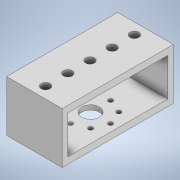
# Autodesk Inventor part: Pièce1
Saved by Autodesk Inventor 2021 (Build 250183000, 183)
## iProperties
Created: 2020-09-01
Part Number: Pièce1
Material: Générique
Document SubType Name: Modeling
Designer: sebas
Density: 1 g/cm^3
Appearance: Par défaut
Author: sebas
Autodesk Inventor part; units mm, degrees
ref_plane "YZ Plane" through (0, 0, 0) normal (1, 0, 0) x (0, 1, 0)
ref_plane "XZ Plane" through (0, 0, 0) normal (0, 1, 0) x (-1, 0, 0)
ref_plane "XY Plane" through (0, 0, 0) normal (0, 0, 1) x (1, 0, 0)
sketch "Esquisse1" plane through (0, 0, 0) normal (0, 1, 0) x (-1, 0, 0)
  line L0 (0, 0) -> (25, 0)
  line L1 (25, 0) -> (25, 50)
  line L2 (25, 50) -> (0, 50)
  line L3 (0, 50) -> (0, 0)
  circle A0 centre (12.25, 25) radius 11
  circle A1 centre (12.25, 25) radius 4
  circle A2 centre (21.25, 25) radius 1
  circle A3 centre (18.614, 31.364) radius 1
  circle A4 centre (12.25, 34) radius 1
  circle A5 centre (5.886, 31.364) radius 1
  circle A6 centre (3.25, 25) radius 1
  circle A7 centre (5.886, 18.636) radius 1
  circle A8 centre (12.25, 16) radius 1
  circle A9 centre (18.614, 18.636) radius 1
  dimension "d0" = 25
  dimension "d1" = 50
  dimension "d2" = 22
  dimension "d3" = 12.75
  dimension "d4" = 25
  dimension "d5" = 8
  dimension "d6" = 2
  dimension "d9" = 360
  dimension "d11" = 4
  dimension "d12" = 18
  constraints: 10 centre point, 8 end point, 2 parallel, 1 coincident, 1 horizontal, 1 perpendicular, 17 other
  measures "d0" distance between parallel lines of L3 L1
  measures "d1" distance between parallel lines of L2 L0
  measures "d2" diameter of A0
  measures "d3" distance from line of L1 A0.centre
  measures "d4" distance from line of A0.centre L0
  measures "d5" diameter of A1
  measures "d6" diameter of A2
  measures "d12" distance of A4.centre A8.centre
extrude "Extrusion1" add sketch "Esquisse1" along normal blind 3 contours L3 L2 L1 L0 | A0
sketch "Esquisse4" plane through (0, 0, 0) normal (0, -1, 0) x (1, 0, 0)
  circle A0 centre (-12.25, 25) radius 11
  circle A1 centre (-12.25, 25) radius 4 projected
  point P0 (0, 0)
  dimension "d17" = 22
  constraints: 1 centre point, 1 coincident
  measures "d17" diameter of A0
extrude "Extrusion2" cut sketch "Esquisse4" against normal blind 1
sketch "Esquisse7" plane through (0, 3, 0) normal (0, 1, 0) x (1, 0, 0)
  line L0 (-25, 0) -> (-25, -50) projected
  line L1 (0, -50) -> (0, 0) projected
  line L2 (-25, 0) -> (0, 0)
  line L3 (0, 0) -> (0, -2.5)
  line L4 (0, -2.5) -> (-25, -2.5)
  line L5 (-25, -2.5) -> (-25, 0)
  dimension "d49" = 2.5
  constraints: 8 end point, 2 parallel, 1 horizontal, 1 perpendicular, 1 point on line
  measures "d49" distance between parallel lines of L2 L4
extrude "Extrusion4" add sketch "Esquisse7" along normal blind 20
sketch "Esquisse8" plane through (0, 3, 0) normal (0, 1, 0) x (1, 0, 0)
  line L0 (0, -50) -> (0, -2.5) projected
  line L1 (-25, -50) -> (0, -50)
  line L2 (0, -50) -> (0, -47.5)
  line L3 (0, -47.5) -> (-25, -47.5)
  line L4 (-25, -47.5) -> (-25, -50)
  point P0 (0, 0)
  dimension "d48" = 2.5
  constraints: 8 end point, 2 parallel, 1 horizontal, 1 perpendicular, 1 point on line
  measures "d48" distance between parallel lines of L3 L1
extrude "Extrusion5" add sketch "Esquisse8" along normal blind 20
sketch "Esquisse9" plane through (0, 3, 47.5) normal (0, 0, -1) x (-1, 0, 0)
  line L0 (0, -3) -> (0, 20) projected
  line L1 (25, 0) -> (25, 20) projected
  line L2 (0, 20) -> (25, 20)
  line L3 (25, 20) -> (25, 17)
  line L4 (25, 17) -> (0, 17)
  line L5 (0, 17) -> (0, 20)
  point P0 (0, 17)
  dimension "d34" = 3
  constraints: 8 end point, 2 parallel, 1 horizontal, 1 perpendicular, 1 point on line
  measures "d34" distance between parallel lines of L4 L2
extrude "Extrusion6" add sketch "Esquisse9" along normal blind 45
sketch "Esquisse10" plane through (0, 23, 0) normal (0, 1, 0) x (1, 0, 0)
  line L0 (0, -50) -> (0, 0) projected
  line L1 (-25, 0) -> (-25, -50) projected
  line L2 (0, 0) -> (-25, 0)
  line L3 (-25, 0) -> (-25, -3)
  line L4 (-25, -3) -> (0, -3)
  line L5 (0, -3) -> (0, 0)
  line L6 (-25, -50) -> (0, -50) projected
  line L7 (0, -50) -> (-25, -50)
  line L8 (-25, -50) -> (-25, -47)
  line L9 (-25, -47) -> (0, -47)
  line L10 (0, -47) -> (0, -50)
  circle A0 centre (-12.5, -5) radius 2
  circle A1 centre (-12.5, -15) radius 2
  circle A2 centre (-12.5, -25) radius 2
  circle A3 centre (-12.5, -35) radius 2
  circle A4 centre (-12.5, -45) radius 2
  dimension "d35" = 4
  dimension "d38" = 10
  dimension "d43" = 3
  dimension "d44" = 3
  dimension "d45" = 2
  constraints: 16 end point, 5 centre point, 4 parallel, 2 horizontal, 2 perpendicular, 2 point on line, 1 vertical, 8 other
  measures "d35" diameter of A0
  measures "d38" distance of A0.centre A1.centre
  measures "d43" distance between parallel lines of L2 L4
  measures "d44" distance between parallel lines of L9 L6
  measures "d45" distance from line of L4 A0.centre
extrude "Extrusion7" cut sketch "Esquisse10" against normal blind 3 contours A0 | A4 | A1 | A2 | A3
